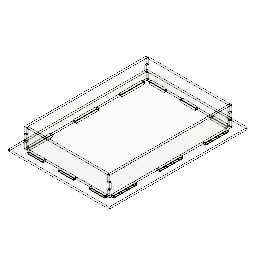
floppyMoldCase_6 (Autodesk Fusion 360 design; units mm, degrees)
Autodesk Fusion 360 part; units mm, degrees
note: some values were not read from the file. Set by a fixed rule: which face or edge a step refers to.
sketch "InitialBottomPlate" plane through (0, 0, 0) normal (0, 0, 1) x (1, 0, 0)
  line L0 (0, 0) -> (125, 0)
  line L1 (125, 0) -> (125, 183)
  line L2 (125, 183) -> (0, 183)
  line L3 (0, 183) -> (0, 0)
  dimension "d84" = 125
  dimension "d85" = 183
  measures "d85" distance of L0.start
extrude "Extrude25" add sketch "InitialBottomPlate" along normal blind 3 makes body 1
extrude "Extrude26" add 1 faces at (41.6667, 0, 1) along direction (0, -1, 0) blind 3 separate body on bodies 1 makes body 2
extrude "Extrude27" add 1 faces at (41.6667, -1, 3) along direction (0, 0, 1) blind 30 separate body on bodies 2 makes body 3
sketch "FrontFingersBotton" plane through (0, 0, 3) normal (0, 0, -1) x (1, 0, 0)
  line L0 (0, 0) -> (125, 0)
  line L1 (125, 3) -> (0, 3)
  line L2 (0, 3) -> (0, 0)
  line L3 (3, 3) -> (3, 0)
  line L4 (26.8, 3) -> (26.8, 0)
  line L5 (50.6, 3) -> (50.6, 0)
  line L6 (74.4, 3) -> (74.4, 0)
  line L7 (98.2, 3) -> (98.2, 0)
  line L8 (122, 3) -> (122, 0)
  line L9 (125, 0) -> (125, 3)
  dimension "d92" = 3
  dimension "d93" = 23.8
  dimension "d96" = 23.8
  dimension "d97" = 0
extrude "Extrude33" add sketch "FrontFingersBotton" along normal blind 3 contours L0 L1 L3 L4 | L0 L1 L5 L6 | L0 L1 L7 L8 bodies 3
sketch "FrontFingerLeft" plane through (0, 0, 0) normal (-1, 0, 0) x (0, -1, 0)
  line L0 (0, 3) -> (3, 3)
  line L1 (3, 3) -> (3, 33)
  line L2 (3, 33) -> (0, 33)
  line L3 (0, 33) -> (0, 3)
  line L4 (0, 23) -> (3, 23)
  line L5 (0, 13) -> (3, 13)
  dimension "d125" = 10
  dimension "d128" = 0
  dimension "d129" = -10
extrude "Extrude38" add sketch "FrontFingerLeft" along normal blind 3 contours L1 L3 L4 L5 bodies 3
sketch "FrontFingerRight" plane through (125, 0, 0) normal (1, 0, 0) x (0, 1, 0)
  line L0 (-3, 3) -> (0, 3)
  line L1 (0, 3) -> (0, 33)
  line L2 (0, 33) -> (-3, 33)
  line L3 (-3, 33) -> (-3, 3)
  line L4 (-3, 23) -> (0, 23)
  line L5 (-3, 13) -> (0, 13)
  dimension "d132" = 10
  dimension "d135" = 0
  dimension "d136" = -10
extrude "Extrude39" add sketch "FrontFingerRight" along normal blind 3 contours L1 L3 L4 L5 bodies 3
extrude "Extrude28" add 1 faces at (125, 61, 1) along direction (1, 0, 0) blind 3 separate body on bodies 1 makes body 4
extrude "Extrude29" add 1 faces at (126, 61, 3) along direction (0, 0, 1) blind 30 separate body on bodies 4 makes body 5
sketch "RightFingersBotton" plane through (0, 0, 3) normal (0, 0, -1) x (1, 0, 0)
  line L0 (125, 0) -> (125, -183)
  line L1 (125, -183) -> (128, -183)
  line L2 (128, -183) -> (128, 0)
  line L3 (128, 0) -> (125, 0)
  line L4 (125, -3) -> (128, -3)
  line L5 (125, -38.4) -> (128, -38.4)
  line L6 (125, -73.8) -> (128, -73.8)
  line L7 (125, -109.2) -> (128, -109.2)
  line L8 (125, -144.6) -> (128, -144.6)
  line L9 (125, -180) -> (128, -180)
  dimension "d106" = 3
  dimension "d107" = 35.4
  dimension "d110" = 0
  dimension "d111" = -35.4
  measures "d106" distance of origin
  measures "d107" distance of origin
extrude "Extrude32" add sketch "RightFingersBotton" along normal blind 3 contours L0 L2 L4 L5 | L0 L2 L6 L7 | L0 L2 L8 L9 bodies 5
sketch "RightFingersFront" plane through (0, 0, 0) normal (0, -1, 0) x (1, 0, 0)
  line L0 (125, 3) -> (128, 3)
  line L1 (128, 3) -> (128, 33)
  line L2 (128, 33) -> (125, 33)
  line L3 (125, 33) -> (125, 3)
  line L4 (125, 23) -> (128, 23)
  line L5 (125, 13) -> (128, 13)
  dimension "d139" = 10
  dimension "d142" = 0
  dimension "d143" = -10
extrude "Extrude40" add sketch "RightFingersFront" along normal blind 3 separate body contours L0 L1 L3 L5 | L1 L2 L3 L4 makes body 6 at (128, -1, 6.3333) makes body 7 at (125, -1, 29.6667)
sketch "RightFingersBack" plane through (0, 183, 0) normal (0, 1, 0) x (-1, 0, 0)
  line L0 (-125, 3) -> (-125, 33)
  line L1 (-125, 33) -> (-128, 33)
  line L2 (-128, 33) -> (-128, 3)
  line L3 (-128, 23) -> (-125, 23)
  line L4 (-128, 13) -> (-125, 13)
  line L5 (-128, 3) -> (-125, 3)
  dimension "d146" = 10
  dimension "d149" = 0
  dimension "d150" = -10
extrude "Extrude41" add sketch "RightFingersBack" along normal blind 3 separate body contours L0 L2 L4 L5 | L0 L1 L2 L3 makes body 8 at (125, 184, 6.3333) makes body 9 at (128, 184, 29.6667)
combine "Combine9" operation add target body 5 tool bodies 9 8 7 6 keep tools
extrude "Extrude34" add 1 faces at (125, 61, 1) along direction (1, 0, 0) blind 15 on bodies 1 bodies 1
extrude "Extrude35" add 1 faces at (93.3333, 183, 1) along direction (0, 1, 0) blind 15 on bodies 1 bodies 1
extrude "Extrude36" add 1 faces at (0, 66, 1) along direction (-1, 0, 0) blind 15 on bodies 1 bodies 1
extrude "Extrude37" add 1 faces at (36.6667, 0, 1) along direction (0, -1, 0) blind 15 on bodies 1 bodies 1
ref_plane "WorkPlane1" through (62.5, 91.5, 1.5) normal (0, -1, 0) x (0, 0, -1)
mirror "Mirror1" about plane through (62.5, 91.5, 1.5) normal (0, -1, 0) of bodies 3 makes body 10
ref_plane "WorkPlane2" through (62.5, 91.5, 1.5) normal (1, 0, 0) x (0, 0, -1)
mirror "Mirror2" about plane through (62.5, 91.5, 1.5) normal (1, 0, 0) of bodies 5 makes body 11
combine "Combine10" operation cut target body 1 tool bodies 10 11 3 5 keep tools
extrude "Extrude42" cut 3 faces at (128, 156.4, 2) (128, 85.6, 2) (128, 14.8, 2) along direction (1, 0, 0) blind 1 on bodies 1 bodies 1
extrude "Extrude43" cut 3 faces at (106.1333, -3, 2) (58.5333, -3, 2) (10.9333, -3, 2) along direction (0, -1, 0) blind 1 on bodies 1 bodies 1
sketch "Sketch21" plane through (129, 0, 0) normal (-1, 0, 0) x (0, -1, 0)
  line L0 (-3, 3) -> (-38.4, 3)
  line L1 (-38.4, 3) -> (-38.4, 0)
  line L2 (-38.4, 0) -> (-3, 0)
  line L3 (-3, 0) -> (-3, 3)
extrude "Extrude44" cut 3 faces at (-3, 14.8, 2) (-3, 85.6, 2) (-3, 156.4, 2) along direction (-1, 0, 0) blind 1 on bodies 1 bodies 1
extrude "Extrude45" cut 3 faces at (10.9333, 186, 2) (58.5333, 186, 2) (106.1333, 186, 2) along direction (0, 1, 0) blind 1 on bodies 1 bodies 1
sketch "BottomExport" plane through (0, 0, 3) normal (0, 0, 1) x (-1, 0, 0)
  line L0 (-140, 15) -> (-140, -198)
  line L1 (-140, -198) -> (15, -198)
  line L2 (15, -198) -> (15, 15)
  line L3 (15, 15) -> (-140, 15)
  line L4 (-3, -183) -> (-3, -187)
  line L5 (-3, -187) -> (-26.8, -187)
  line L6 (-26.8, -187) -> (-26.8, -183)
  line L7 (-26.8, -183) -> (-3, -183)
  line L8 (-50.6, -183) -> (-50.6, -187)
  line L9 (-50.6, -187) -> (-74.4, -187)
  line L10 (-74.4, -187) -> (-74.4, -183)
  line L11 (-74.4, -183) -> (-50.6, -183)
  line L12 (-98.2, -183) -> (-98.2, -187)
  line L13 (-98.2, -187) -> (-122, -187)
  line L14 (-122, -187) -> (-122, -183)
  line L15 (-122, -183) -> (-98.2, -183)
  line L16 (0, -144.6) -> (4, -144.6)
  line L17 (4, -144.6) -> (4, -180)
  line L18 (4, -180) -> (0, -180)
  line L19 (0, -180) -> (0, -144.6)
  line L20 (0, -73.8) -> (4, -73.8)
  line L21 (4, -73.8) -> (4, -109.2)
  line L22 (4, -109.2) -> (0, -109.2)
  line L23 (0, -109.2) -> (0, -73.8)
  line L24 (0, -3) -> (4, -3)
  line L25 (4, -3) -> (4, -38.4)
  line L26 (4, -38.4) -> (0, -38.4)
  line L27 (0, -38.4) -> (0, -3)
  line L28 (-26.8, 0) -> (-26.8, 4)
  line L29 (-26.8, 4) -> (-3, 4)
  line L30 (-3, 4) -> (-3, 0)
  line L31 (-3, 0) -> (-26.8, 0)
  line L32 (-74.4, 0) -> (-74.4, 4)
  line L33 (-74.4, 4) -> (-50.6, 4)
  line L34 (-50.6, 4) -> (-50.6, 0)
  line L35 (-50.6, 0) -> (-74.4, 0)
  line L36 (-122, 0) -> (-122, 4)
  line L37 (-122, 4) -> (-98.2, 4)
  line L38 (-98.2, 4) -> (-98.2, 0)
  line L39 (-98.2, 0) -> (-122, 0)
  line L40 (-129, -3) -> (-125, -3)
  line L41 (-125, -3) -> (-125, -38.4)
  line L42 (-125, -38.4) -> (-129, -38.4)
  line L43 (-129, -38.4) -> (-129, -3)
  line L44 (-129, -144.6) -> (-125, -144.6)
  line L45 (-125, -144.6) -> (-125, -180)
  line L46 (-125, -180) -> (-129, -180)
  line L47 (-129, -180) -> (-129, -144.6)
  line L48 (-129, -73.8) -> (-125, -73.8)
  line L49 (-125, -73.8) -> (-125, -109.2)
  line L50 (-125, -109.2) -> (-129, -109.2)
  line L51 (-129, -109.2) -> (-129, -73.8)
sketch "FrontBackExport" plane through (0, -3, 0) normal (0, -1, 0) x (1, 0, 0)
  line L0 (122, 3) -> (125, 3)
  line L1 (125, 3) -> (125, 13)
  line L2 (125, 13) -> (128, 13)
  line L3 (128, 13) -> (128, 23)
  line L4 (128, 23) -> (125, 23)
  line L5 (125, 23) -> (125, 33)
  line L6 (125, 33) -> (0, 33)
  line L7 (0, 33) -> (0, 23)
  line L8 (0, 23) -> (-3, 23)
  line L9 (-3, 23) -> (-3, 13)
  line L10 (-3, 13) -> (0, 13)
  line L11 (0, 13) -> (0, 3)
  line L12 (0, 3) -> (3, 3)
  line L13 (3, 3) -> (3, 0)
  line L14 (3, 0) -> (26.8, 0)
  line L15 (26.8, 0) -> (26.8, 3)
  line L16 (26.8, 3) -> (50.6, 3)
  line L17 (50.6, 3) -> (50.6, 0)
  line L18 (50.6, 0) -> (74.4, 0)
  line L19 (74.4, 0) -> (74.4, 3)
  line L20 (74.4, 3) -> (98.2, 3)
  line L21 (98.2, 3) -> (98.2, 0)
  line L22 (98.2, 0) -> (122, 0)
  line L23 (122, 0) -> (122, 3)
sketch "LeftRightExport" plane through (128, 0, 0) normal (1, 0, 0) x (0, 1, 0)
  line L0 (180, 3) -> (186, 3)
  line L1 (186, 3) -> (186, 13)
  line L2 (186, 13) -> (183, 13)
  line L3 (183, 13) -> (183, 23)
  line L4 (183, 23) -> (186, 23)
  line L5 (186, 23) -> (186, 33)
  line L6 (186, 33) -> (-3, 33)
  line L7 (-3, 33) -> (-3, 23)
  line L8 (-3, 23) -> (0, 23)
  line L9 (0, 23) -> (0, 13)
  line L10 (0, 13) -> (-3, 13)
  line L11 (-3, 13) -> (-3, 3)
  line L12 (-3, 3) -> (3, 3)
  line L13 (3, 3) -> (3, 0)
  line L14 (3, 0) -> (38.4, 0)
  line L15 (38.4, 0) -> (38.4, 3)
  line L16 (38.4, 3) -> (73.8, 3)
  line L17 (73.8, 3) -> (73.8, 0)
  line L18 (73.8, 0) -> (109.2, 0)
  line L19 (109.2, 0) -> (109.2, 3)
  line L20 (109.2, 3) -> (144.6, 3)
  line L21 (144.6, 3) -> (144.6, 0)
  line L22 (144.6, 0) -> (180, 0)
  line L23 (180, 0) -> (180, 3)
hidden bodies 2 4 6 7 8 9
equation "thickness = 3 mm" comment "Material/Plate thickness"
equation "height = 30 mm"
equation "border = 15 mm"
equation "width = 125 mm" comment "inside mold width"
equation "length = 183 mm" comment "inside mold length"
equation "d84 = width"
equation "d85 = length"
equation "d86 = thickness"
equation "d88 = thickness"
equation "d90 = height"
equation "d92 = thickness"
equation "d93 = ( width - thickness * 2 ) / 5"
equation "d96 = ( width - thickness - thickness ) / 5"
equation "d98 = thickness"
equation "d100 = height"
equation "d106 = thickness"
equation "d107 = ( length - thickness - thickness ) / 5"
equation "d111 = -( length - thickness - thickness ) / 5"
equation "d112 = thickness"
equation "d114 = thickness"
equation "d116 = border"
equation "d118 = border"
equation "d120 = border"
equation "d122 = border"
equation "d125 = height / 3"
equation "d129 = -( height / 3 )"
equation "d130 = thickness"
equation "d132 = height / 3"
equation "d136 = -( height / 3 )"
equation "d137 = thickness"
equation "d139 = height / 3"
equation "d143 = -( height / 3 )"
equation "d144 = thickness"
equation "d146 = height / 3"
equation "d150 = -( height / 3 )"
equation "d151 = thickness"
named bodies: "BottomPlate", "TempFront", "Front", "TempRight", "Right", "Back (Mirror)", "TempRightFingerFront1", "TempRightFingerFront2", "TempRightFingerBack1", "TempRightFingerBack2", "Left (Mirror)"
